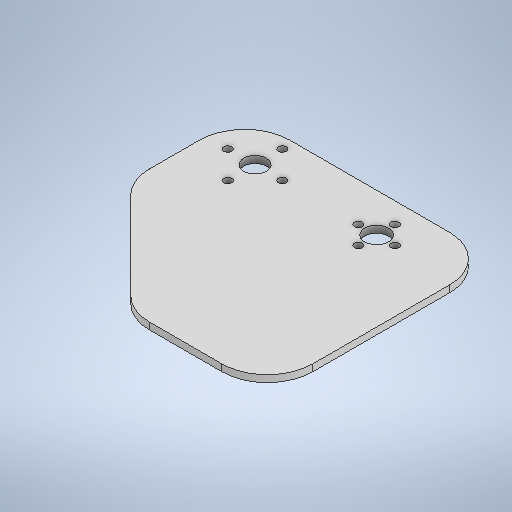
# Autodesk Inventor part: TopMount
Saved by Autodesk Inventor 2025.2 (Build 292293000, 293)
## iProperties
Created: 2025-07-18
Part Number: TopMount
Material: Generic
Document SubType Name: Modeling
Designer: Simon
Density: 1 g/cm^3
Appearance: Default
Author: Simon
Autodesk Inventor part; units mm, degrees
ref_plane "YZ Plane" through (0, 0, 0) normal (1, 0, 0) x (0, 1, 0)
ref_plane "XZ Plane" through (0, 0, 0) normal (0, 1, 0) x (-1, 0, 0)
ref_plane "XY Plane" through (0, 0, 0) normal (0, 0, 1) x (1, 0, 0)
sketch "Sketch1" plane through (0, 0, 0) normal (0, 1, 0) x (-1, 0, 0)
  line L0 (-75, 25) -> (75, 25)
  line L1 (75, 25) -> (75, -25)
  line L2 (75, -25) -> (-75, -25)
  line L3 (-75, -25) -> (-75, 25)
  line L4 (-75, 25) -> (75, -25) construction
  line L5 (75, 25) -> (-75, -25) construction
  line L6 (-75, -25) -> (-35, -25)
  line L7 (-35, -25) -> (-35, 25)
  line L8 (-35, 25) -> (-75, 25)
  line L9 (-75, 25) -> (-75, -25)
  line L10 (-35, 25) -> (-35, 75)
  line L11 (-35, 75) -> (75, 75)
  line L12 (75, 75) -> (75, 25)
  line L13 (-35, 75) -> (25, 75)
  line L14 (25, 75) -> (75, 25)
  point P0 (0, 0)
  point P1 (-35, -25)
  dimension "d0" = 150
  dimension "d1" = 50
  dimension "d57" = 40
  dimension "d58" = 50
  dimension "d59" = 50
  dimension "d60" = 60
  constraints: 30 end point, 5 perpendicular, 4 parallel, 3 point on line, 2 horizontal, 2 midpoint
  measures "d0" distance of L1.end L2.end
  measures "d1" distance of L0.end L1.end
  measures "d57" distance of L8.end L7.end
  measures "d58" distance of L7.end L10.end
  measures "d59" distance of L11.end L0.end
  measures "d60" distance of L10.end L13.end
extrude "Extrusion1" add sketch "Sketch1" along normal blind 3 contours L10 L11 L14 L0 | L0 L1 L2 L7
sketch "Sketch6" plane through (0, 3, 0) normal (0, 1, 0) x (1, 0, 0)
  line L0 (35, 25) -> (-75, 25) projected
  line L1 (0, 25) -> (0, 8)
  circle A0 centre (0, 8) radius 5.25
  line L2 (0, 8) -> (-53.4, 8)
  circle A1 centre (-53.4, 8) radius 5
  circle A2 centre (0, 8) radius 8
  circle A3 centre (0, 16) radius 1.75
  circle A4 centre (-8, 8) radius 1.75
  circle A5 centre (0, 0) radius 1.75
  circle A6 centre (8, 8) radius 1.75
  circle A7 centre (-53.4, 8) radius 12
  line L3 (-53.4, -4) -> (-53.4, 20)
  circle A8 centre (-53.4, 20) radius 1.75
  circle A9 centre (-65.4, 8) radius 1.75
  circle A10 centre (-53.4, -4) radius 1.75
  circle A11 centre (-41.4, 8) radius 1.75
  point P0 (0, 0)
  point P1 (75, 25)
  dimension "d49" = 24
  dimension "d40" = 17
  dimension "d41" = 10.5
  dimension "d42" = 53.4
  dimension "d43" = 10
  dimension "d44" = 3.5
  dimension "d47" = 360
  dimension "d50" = 3.5
  dimension "d53" = 360
  constraints: 11 centre point, 6 end point, 5 coincident, 2 point on circle, 2 point on line, 2 vertical, 1 horizontal, 1 midpoint, 1 vertical alignment, 20 other
  measures "d40" distance of L1.start L1.end
  measures "d41" diameter of A0
  measures "d42" distance of L2.start L2.end
  measures "d43" diameter of A1
  measures "d44" diameter of A3
  measures "d50" diameter of A8
extrude "Extrusion6" cut sketch "Sketch6" against normal through all contours A3 A2 L1 | A11 A7 L2 | L2 A7 A11 | L1 A2 A3 | A2 A3 L1 | L1 A3 A2 | A4 L2 A2 | A2 L2 A4 | A0 L2 L1 | L1 L2 A0 | A6 A2 | A2 A6 | A2 A4 L2 | L2 A4 A2 | A5 A2 | A2 A5 | A7 A11 L2 | L2 A11 A7 | A8 L3 A7 | A7 A8 | A10 A7 | A7 L3 A10 | A1 L3 L2 | L2 L3 A1 | L3 A8 A7 | A7 A10 L3 | L3 A1 | A9 A7 | A7 A9
fillet "Fillet1" radius 20 5 edges at (35, 1.5, -25) (35, 1.5, 75) (-25, 1.5, 75) (-75, 1.5, 25) (-75, 1.5, -25)
body "Solid1"
